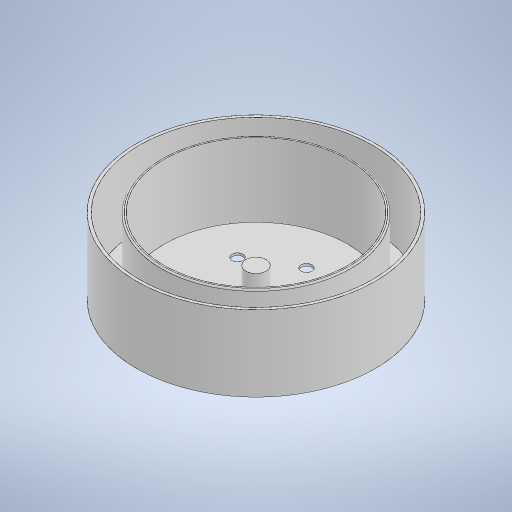
# Autodesk Inventor part: Mold - Wheel
Saved by Autodesk Inventor 2023.2 (Build 272271000, 271)
## iProperties
Created: 2023-09-22
Part Number: Mold - Wheel
Material: Generic
Document SubType Name: Modeling
Designer: Nathan Cai
Density: 1 g/cm^3
Appearance: Default
Author: Nathan Cai
Autodesk Inventor part; units mm, degrees
ref_plane "YZ Plane" through (0, 0, 0) normal (1, 0, 0) x (0, 1, 0)
ref_plane "XZ Plane" through (0, 0, 0) normal (0, 1, 0) x (-1, 0, 0)
ref_plane "XY Plane" through (0, 0, 0) normal (0, 0, 1) x (1, 0, 0)
sketch "Sketch1" plane through (0, 0, 0) normal (0, 1, 0) x (-1, 0, 0)
  circle A0 centre (0, 0) radius 41.275
  dimension "d0" = 82.55
  constraints: 1 centre point, 1 coincident
  measures "d0" diameter of A0
extrude "Extrusion1" add sketch "Sketch1" along normal blind 0.75
sketch "Sketch2" plane through (0, 0.75, 0) normal (0, 1, 0) x (1, 0, 0)
  circle A0 centre (0, 0) radius 31.75
  circle A1 centre (0, 0) radius 41.275 projected
  circle A2 centre (0, 0) radius 32.75
  circle A3 centre (0, 0) radius 40.275
  dimension "d3" = 63.5
  dimension "d4" = 1
  dimension "d5" = 1
  constraints: 3 centre point, 1 coincident
  measures "d3" diameter of A0
  measures "d4" radial gap between concentric circles of A0 A2
  measures "d5" radial gap between concentric circles of A1 A3
extrude "Extrusion2" add sketch "Sketch2" along normal blind 25.4
fillet "Fillet1" radius 0.5 1 edges at (-32.75, 26.15, 0)
sketch "Sketch3" plane through (0, 0.75, 0) normal (0, 1, 0) x (1, 0, 0)
  circle A0 centre (0, 0) radius 17.4625 construction
  line L0 (0, 0) -> (0, -17.4625) construction
  circle A1 centre (0, -17.4625) radius 1.905
  circle A2 centre (15.123, -8.7313) radius 1.905
  circle A3 centre (15.123, 8.7312) radius 1.905
  circle A4 centre (0, 17.4625) radius 1.905
  circle A5 centre (-15.123, 8.7313) radius 1.905
  circle A6 centre (-15.123, -8.7312) radius 1.905
  dimension "d9" = 34.925
  dimension "d10" = 3.81
  dimension "d13" = 360
  constraints: 6 centre point, 2 coincident, 2 end point, 1 vertical, 1 vertical alignment, 15 other
  measures "d10" diameter of A1
extrude "Extrusion3" cut sketch "Sketch3" against normal through all
sketch "Sketch4" plane through (0, 0.75, 0) normal (0, 1, 0) x (1, 0, 0)
  circle A0 centre (0, 0) radius 3.4925
  dimension "d17" = 6.985
  constraints: 1 centre point, 1 coincident
  measures "d17" diameter of A0
extrude "Extrusion4" add sketch "Sketch4" along normal blind 9.525
body "Solid1"
